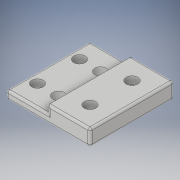
# Autodesk Inventor part: syringepumpplate
Saved by Autodesk Inventor 2018 (Build 220112000, 112)
## iProperties
Created: 2018-10-04
Part Number: syringepumpplate
Material: Generic
Document SubType Name: Modeling
Designer: Iek Man Lei
Density: 1 g/cm^3
Appearance: Default
Author: Iek Man Lei
Autodesk Inventor part; units mm, degrees
ref_plane "YZ Plane" through (0, 0, 0) normal (1, 0, 0) x (0, 1, 0)
ref_plane "XZ Plane" through (0, 0, 0) normal (0, 1, 0) x (-1, 0, 0)
ref_plane "XY Plane" through (0, 0, 0) normal (0, 0, 1) x (1, 0, 0)
sketch "Sketch1" plane through (0, 0, 0) normal (0, 1, 0) x (-1, 0, 0)
  line L0 (17.7143, 25.1429) -> (-22.2857, 25.1429)
  line L1 (-22.2857, 25.1429) -> (-22.2857, -14.8571)
  line L2 (-22.2857, -14.8571) -> (17.7143, -14.8571)
  line L3 (17.7143, -14.8571) -> (17.7143, 25.1429)
  circle A0 centre (12.7143, 15.1429) radius 2.75
  circle A1 centre (12.7143, -4.8571) radius 2.75
  circle A2 centre (2.7143, -4.8571) radius 2.75
  circle A3 centre (2.7143, 15.1429) radius 2.75
  circle A4 centre (-12.2857, 15.1429) radius 2.75
  circle A5 centre (-12.2857, -4.8571) radius 2.75
  point P0 (0, 0)
  dimension "d1" = 40
  dimension "d2" = 5.5
  dimension "d3" = 5.5
  dimension "d4" = 5.5
  dimension "d5" = 5.5
  dimension "d6" = 5.5
  dimension "d7" = 5.5
  dimension "d9" = 10
  dimension "d12" = 20
  dimension "d13" = 10
  dimension "d17" = 5
  dimension "d28" = 10
  dimension "d32" = 15
  constraints: 8 end point, 6 centre point, 3 horizontal alignment, 3 vertical alignment, 2 parallel, 1 horizontal, 1 perpendicular
  measures "d1" distance of L0.end L1.end
  measures "d2" diameter of A0
  measures "d3" diameter of A1
  measures "d4" diameter of A2
  measures "d5" diameter of A3
  measures "d6" diameter of A4
  measures "d7" diameter of A5
  measures "d9" distance of A2.centre A1.centre
  measures "d12" distance of A4.centre A5.centre
  measures "d13" distance from line of L2 A5.centre
  measures "d17" distance from line of L3 A1.centre
  measures "d28" distance from line of L1 A5.centre
  measures "d32" distance of A5.centre A2.centre
extrude "Extrusion1" add sketch "Sketch1" along normal blind 4
sketch "Sketch2" plane through (0, 4, 0) normal (0, 1, 0) x (1, 0, 0)
  line L0 (22.2857, -25.1429) -> (22.2857, 14.8571) projected
  line L1 (22.2857, 14.8571) -> (2.2857, 14.8571)
  line L2 (2.2857, 14.8571) -> (2.2857, -25.1429)
  line L3 (2.2857, -25.1429) -> (22.2857, -25.1429)
  line L4 (22.2857, -25.1429) -> (22.2857, 14.8571)
  point P0 (0, 0)
  dimension "d30" = 20
  dimension "d31" = 40
  constraints: 8 end point, 2 parallel, 1 horizontal, 1 perpendicular
  measures "d30" distance of L0.end L1.end
  measures "d31" distance of L1.end L2.end
extrude "Extrusion2" add sketch "Sketch2" along normal blind 3.7
sketch "Sketch3" plane through (12.2857, 4, -4.8571) normal (0, -1, 0) x (1, 0, 0)
  circle A0 centre (0, 0) radius 2.7975
  circle A1 centre (0, 20) radius 2.75
  line L0 (10, -10) -> (-30, -10) projected
  line L1 (10, 30) -> (10, -10) projected
  point P0 (-12.2857, 4.8571)
  dimension "d21" = 20
  dimension "d22" = 5.5
  dimension "d23" = 10
  dimension "d24" = 10
  constraints: 2 centre point, 1 vertical alignment
  measures "d21" distance of A1.centre A0.centre
  measures "d22" diameter of A1
  measures "d23" distance from line of L0 A0.centre
  measures "d24" distance from line of L1 A0.centre
extrude "Extrusion3" cut sketch "Sketch3" against normal blind 3.7
fillet "Fillet2" radius 1 16 edges at (2.2857, 0, 25.1429) (-7.7143, 4, 25.1429) (12.2857, 7.7, 25.1429) (22.2857, 3.85, 25.1429) (22.2857, 7.7, 5.1429) (12.2857, 7.7, -14.8571) (-17.7143, 4, 5.1429) (-7.7143, 4, -14.8571) (2.2857, 0, -14.8571) (-17.7143, 2, -14.8571) (-17.7143, 0, 5.1429) (-17.7143, 2, 25.1429) (22.2857, 3.85, -14.8571) (22.2857, 0, 5.1429) (2.2857, 5.85, 25.1429) (2.2857, 5.85, -14.8571)
body "Solid1"
